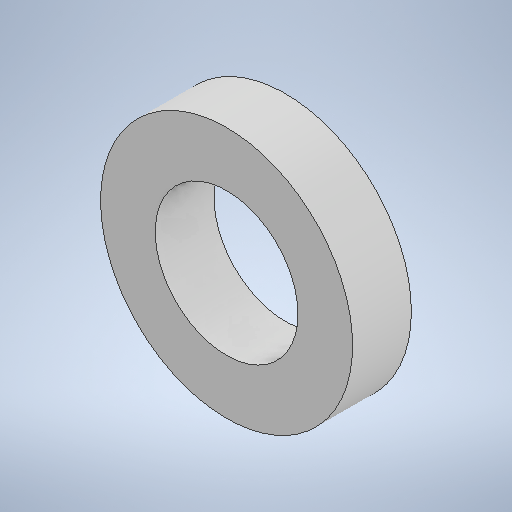
# Autodesk Inventor part: Part3
Saved by Autodesk Inventor 2025.2 (Build 292293000, 293)
## iProperties
Created: 2024-12-14
Part Number: Part3
Material: 一般
Document SubType Name: Modeling
Designer: mahhy
Density: 1 g/cm^3
Appearance: 既定
Author: mahhy
Autodesk Inventor part; units mm, degrees
ref_plane "YZ Plane" through (0, 0, 0) normal (1, 0, 0) x (0, 1, 0)
ref_plane "XZ Plane" through (0, 0, 0) normal (0, 1, 0) x (-1, 0, 0)
ref_plane "XY Plane" through (0, 0, 0) normal (0, 0, 1) x (1, 0, 0)
sketch "スケッチ4" plane through (0, 0, 0) normal (0, 0, 1) x (1, 0, 0)
  circle A0 centre (0, 0) radius 15
  circle A1 centre (0, 0) radius 8.5
  dimension "d8" = 30
  dimension "d9" = 17
  constraints: 2 centre point, 2 coincident
  measures "d8" diameter of A0
  measures "d9" diameter of A1
extrude "押し出し3" add sketch "スケッチ4" against normal blind 7
